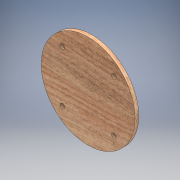
# Autodesk Inventor part: base
Saved by Autodesk Inventor 2017.3 (Build 213256000, 256)
## iProperties
Part Number: base
Material: Bois (bouleau)
Document SubType Name: Modeling
Designer: Piou piou
Density: 0.55 g/cm^3
Appearance: Bouleau - Poli naturel
Mass: 136.848 g
Surface Area: 682.354 cm^2
Volume: 248.814 cm^3
Author: Piou piou
Autodesk Inventor part; units mm, degrees
ref_plane "YZ Plane" through (0, 0, 0) normal (1, 0, 0) x (0, 1, 0)
ref_plane "XZ Plane" through (0, 0, 0) normal (0, 1, 0) x (-1, 0, 0)
ref_plane "XY Plane" through (0, 0, 0) normal (0, 0, 1) x (1, 0, 0)
sketch "Esquisse1" plane through (0, 0, 0) normal (0, 1, 0) x (-1, 0, 0)
  circle A0 centre (0, 0) radius 100
  line L0 (55, -55) -> (-55, -55)
  line L1 (-55, -55) -> (-55, 55)
  line L2 (-55, 55) -> (55, 55)
  line L3 (55, 55) -> (55, -55)
  line L4 (55, -55) -> (-55, 55) construction
  line L5 (-55, -55) -> (55, 55) construction
  circle A1 centre (-55, 55) radius 5
  circle A2 centre (55, 55) radius 5
  circle A3 centre (55, -55) radius 5
  circle A4 centre (-55, -55) radius 5
  dimension "d0" = 200
  dimension "d3" = 110
  dimension "d4" = 10
  constraints: 12 end point, 5 centre point, 5 coincident, 3 equal radius, 2 midpoint, 2 parallel, 2 perpendicular, 1 horizontal
  measures "d0" diameter of A0
  measures "d3" distance of L0.end L1.end
  measures "d4" diameter of A1
extrude "Extrusion1" add sketch "Esquisse1" along normal blind 8 contours A0 | A4 L1 L0 | A4 L1 A1 L2 A2 L3 A3 L0 | L0 L1 A4 | A3 L3 L0 | L0 L3 A3 | A1 L2 L1 | L1 L2 A1 | A2 L2 L3 | L3 L2 A2
sketch "Esquisse2" plane through (0, 0, 0) normal (0, -1, 0) x (1, 0, 0)
  line L0 (-55, -55) -> (55, -55)
  line L1 (55, -55) -> (55, 55)
  line L2 (55, 55) -> (-55, 55)
  line L3 (-55, 55) -> (-55, -55)
  line L4 (-55, -55) -> (55, 55) construction
  line L5 (55, -55) -> (-55, 55) construction
  circle A0 centre (-55, 55) radius 5
  circle A1 centre (55, 55) radius 5
  circle A2 centre (55, -55) radius 5
  circle A3 centre (-55, -55) radius 5
  point P0 (0, 0)
  dimension "d5" = 110
  dimension "d6" = 10
  constraints: 12 end point, 4 centre point, 4 coincident, 3 equal radius, 2 midpoint, 2 parallel, 2 perpendicular, 1 horizontal
  measures "d5" distance of L0.end L1.end
  measures "d6" diameter of A0
extrude "Extrusion2" cut sketch "Esquisse2" against normal blind 10 contours L3 A3 L0 | L0 A3 L3 | A2 L1 L0 | L0 L1 A2 | A0 L2 L3 | L3 L2 A0 | A1 L2 L1 | L1 L2 A1
